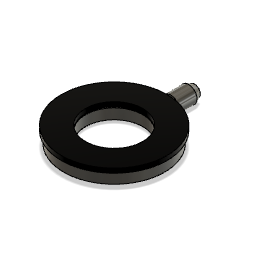
Assembly v4 (Autodesk Fusion 360 archive; units mm, degrees)
design "Polarizer"
Autodesk Fusion 360 part; units mm, degrees
sketch "Sketch1" plane through (0, 0, 0) normal (0, 1, 0) x (1, 0, 0)
  circle A0 centre (0, 0) radius 37.95
  dimension "d1" = 75.9
  constraint coincident A0.centre origin
  measures "d1" diameter of A0
extrude "Extrude1" add sketch "Sketch1" along normal blind 7.8 makes body 1
sketch "Sketch2" plane through (0, 7.8, 0) normal (0, 1, 0) x (-1, 0, 0)
  circle A0 centre (0, 0) radius 37.95
  circle A1 centre (0, 0) radius 21.55
  dimension "d4" = 43.1
  constraint concentric A0 A1
  measures "d4" diameter of A1
extrude "Extrude2" cut sketch "Sketch2" against normal blind 60 contours A1 bodies 1
sketch "Sketch3" plane through (0, 7.8, 0) normal (0, 1, 0) x (-1, 0, 0)
  circle A0 centre (0, 0) radius 21.55
  circle A1 centre (0, 0) radius 37.95
  circle A2 centre (0, 0) radius 39.75
  dimension "d7" = 79.5
  constraint coincident A0.centre A1.centre
  measures "d7" diameter of A2
extrude "Extrude3" add sketch "Sketch3" along normal blind 3.3 separate body contours A1 | A2 makes body 2
ref_plane "WorkPlane1" through (0, 2.0555, -21.55) normal (0, 0, 1) x (1, 0, 0)
ref_plane "WorkPlane2" through (0, 2.0555, -36.55) normal (0, 0, 1) x (1, 0, 0)
split "Split1" by plane through (0, 2.0555, -36.55) normal (0, 0, 1) bodies 1 makes body 3 at (-0.5368, 0, -31.5299)
sketch "Sketch6" plane through (0, 0, -36.55) normal (0, 0, -1) x (-1, 0, 0)
  line L0 (-10.2127, 7.8) -> (-10.2127, 0)
  line L1 (-10.2127, 0) -> (10.2127, 0)
  line L2 (10.2127, 0) -> (10.2127, 7.8)
  line L3 (10.2127, 7.8) -> (-10.2127, 7.8)
  line L4 (0, 0) -> (0, 7.8)
  circle A0 centre (0, 3.9) radius 4.75
  circle A1 centre (0, 3.9) radius 6.35
  dimension "d14" = 9.5
  dimension "d15" = 12.7
  constraint coincident L4.start origin
  constraint midpoint L3 L4.end
  constraint midpoint L4 A0.centre
  constraint concentric A0 A1
  measures "d14" diameter of A0
  measures "d15" diameter of A1
extrude "Extrude4" add sketch "Sketch6" along normal blind 24 contours L3 A0 | L1 L3 L4 A0 | L1 A0 | L1 L3 L4 A0 bodies 3
extrude "Extrude5" add sketch "Sketch6" along normal blind 19.1 from surface at 4.9 contours L3 A0 A1 | L1 L3 A0 A1 | L1 A0 A1 | L1 L3 A0 A1 bodies 3
chamfer "Chamfer1" distance 2 distance2 4.5 1 edges at (5.9203, 1.6037, -60.55) measured on face at (-0.0223, 5.1092, -60.55) on bodies 3
chamfer "Chamfer2" distance 1 distance2 1 1 edges at (5.9203, 1.6037, -41.45) measured on face at (-6.3184, 4.5323, -51.1833) on bodies 3
copy_body "Body->Comp1" bodies 2 removing the originals makes body 4 in component "Ring"
copy_body "Body->Comp2" bodies 3 removing the originals makes body 5 in component "Base"
component "Ring" placed x (1, 0, 0) y (0, 1, 0) z (0, 0, 1) at (0, 0.7, 0)
component "Base" placed x (1, 0, 0) y (0, 1, 0) z (0, 0, 1) at (0, 0, 0)
hidden bodies 1

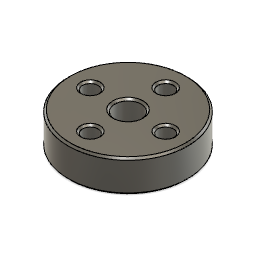
design "Mount"
Autodesk Fusion 360 part; units mm, degrees
sketch "Sketch1" plane through (0, 0, 0) normal (0, 1, 0) x (1, 0, 0)
  circle A0 centre (0, 0) radius 9.5
  circle A1 centre (0, 0) radius 2.1
  circle A2 centre (6, 0) radius 1.25
  circle A3 centre (0, 0) radius 6 construction
  circle A4 centre (0, 6) radius 1.25
  circle A5 centre (-6, 0) radius 1.25
  circle A6 centre (0, -6) radius 1.25
  dimension "d1" = 19
  dimension "d2" = 4.2
  dimension "d3" = 2.5
  dimension "d5" = 360
  constraint coincident A0.centre A1.centre
  constraint concentric A0 A1
  constraint concentric A0 A3
  constraint coincident A2.centre A3
  measures "d1" diameter of A0
  measures "d2" diameter of A1
  measures "d3" diameter of A2
extrude "Extrude1" add sketch "Sketch1" along normal blind 5.1
chamfer "Chamfer1" distance 0.3 angle 45 2 edges at (-8.8571, 5.1, 3.4353) (-8.8571, 0, 3.4353)
chamfer "Chamfer2" distance 0.3 angle 45 10 edges at (-1.9579, 5.1, -0.7594) (-1.1654, 5.1, -6.452) (-7.1654, 5.1, -0.452) (-1.1654, 5.1, 5.548) (4.8346, 5.1, -0.452) (-1.1654, 0, 5.548) (-7.1654, 0, -0.452) (-1.1654, 0, -6.452) (-1.9579, 0, -0.7594) (4.8346, 0, -0.452)
